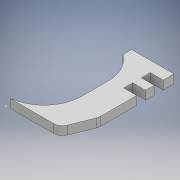
# Autodesk Inventor part: Finger
Saved by Autodesk Inventor 2017 (Build 210142000, 142)
## iProperties
Created: 2017-05-09
Part Number: Finger
Material: Generic
Document SubType Name: Modeling
Designer: s4461999
Density: 1 g/cm^3
Appearance: Default
Author: s4461999
Autodesk Inventor part; units mm, degrees
ref_plane "YZ Plane" through (0, 0, 0) normal (1, 0, 0) x (0, 1, 0)
ref_plane "XZ Plane" through (0, 0, 0) normal (0, 1, 0) x (-1, 0, 0)
ref_plane "XY Plane" through (0, 0, 0) normal (0, 0, 1) x (1, 0, 0)
sketch "Sketch1" plane through (0, 0, 0) normal (0, 0, 1) x (1, 0, 0)
  arc A0 (6.0987, 0.8622) -> (22, 22) centre (0, 22) ccw
  line L0 (22, 22) -> (22, 37)
  arc A1 (22, 37) -> (13, 54.7482) centre (0, 37) ccw
  line L1 (13, 54.7482) -> (13, 66.7482)
  line L2 (22.5, 90) -> (22.5, 66.7482)
  line L3 (22.5, 90) -> (37.5, 90)
  line L4 (13, 66.7482) -> (22.5, 66.7482)
  line L5 (2.6116, 0) -> (27.6759, 0)
  line L6 (32.3216, 3.1515) -> (37.1457, 15.2755)
  arc A2 (37.1457, 15.2755) -> (37.5, 17.1241) centre (32.5, 17.1241) ccw
  arc A3 (27.6759, 0) -> (32.3216, 3.1515) centre (27.6759, 5) ccw
  line L7 (37.5, 53.562) -> (30, 53.562)
  line L8 (30, 53.562) -> (30, 48.362)
  line L9 (30, 48.362) -> (37.5, 48.362)
  line L10 (37.5, 43.362) -> (30, 43.362)
  line L11 (30, 43.362) -> (30, 38.162)
  line L12 (30, 38.162) -> (37.5, 38.162)
  line L13 (37.5, 90) -> (37.5, 53.562)
  line L14 (37.5, 48.362) -> (37.5, 43.362)
  line L15 (37.5, 38.162) -> (37.5, 17.1241)
  line L16 (6.0987, 0.8622) -> (2.6116, 0)
  point P0 (0, 0)
  dimension "d0" = 22
  dimension "d1" = 90
  dimension "d2" = 0
  dimension "d3" = 15
  dimension "d4" = 0
  dimension "d5" = 13
  dimension "d6" = 22
  dimension "d7" = 12
  dimension "d8" = 22.5
  dimension "d10" = 90
  dimension "d11" = 37
  dimension "d12" = 5
  dimension "d13" = 12.1241
  dimension "d14" = 5.2
  dimension "d15" = 5.2
  dimension "d16" = 5
  constraints: 34 end point, 8 point on circle, 7 perpendicular, 6 tangent, 6 vertical, 4 centre point, 4 horizontal, 2 point on line, 1 equal radius, 1 parallel
  measures "d0" radius of A0
  measures "d2" horizontal distance of point (0, 0) A0.centre
  measures "d3" distance of L0.start L0.end
  measures "d4" horizontal distance of point (0, 0) A1.centre
  measures "d5" horizontal distance of A1.centre L1.start
  measures "d6" radius of A1
  measures "d7" distance of L1.start L1.end
  measures "d8" distance from line of point (0, 0) L2
  measures "d10" distance from line of point (0, 0) L3
  measures "d11" distance from line of L6 A0.centre
  measures "d12" radius of A2
  measures "d13" vertical distance of L6.start L6.end
  measures "d14" distance between parallel lines of L9 L7
  measures "d15" distance between parallel lines of L12 L10
  measures "d16" distance between parallel lines of L9 L10
sketch "Sketch2" plane through (0, 0, 0) normal (0, 0, 1) x (1, 0, 0)
  point P0 (0, 0)
extrude "Extrusion1" add sketch "Sketch1" along normal blind 5
sketch "Sketch3" plane through (0, 0, 5) normal (0, 0, 1) x (1, 0, 0)
  line L0 (22.5, 90) -> (22.5, 66.7482) projected
  line L1 (37.5, 90) -> (22.5, 90) projected
  point P0 (0, 0)
  point P1 (30, 86.5)
  point P2 (30, 68.5)
  dimension "d20" = 18
  dimension "d21" = 7.5
  dimension "d22" = 7.5
  dimension "d23" = 3.5
  measures "d20" distance of point (30, 68.5) point (30, 86.5)
  measures "d21" distance from line of point (30, 86.5) L0
  measures "d22" distance from line of L0 point (30, 68.5)
  measures "d23" distance from line of L1 point (30, 86.5)
hole "Hole1" at (30, 86.5, 5) at (30, 68.5, 5) direction (0, 0, -1) diameter 3.4 end through all
sketch "Sketch4" plane through (22.5, 66.7482, 0) normal (-1, 0, 0) x (0, 0, 1)
  line L0 (-7.9102, 0) -> (13.3435, 0)
  line L1 (13.3435, 0) -> (13.3435, 24.2425)
  line L2 (13.3435, 24.2425) -> (-7.9102, 24.2425)
  line L3 (-7.9102, 24.2425) -> (-7.9102, 0)
  line L4 (0, 0) -> (5, 0) projected
  point P0 (0, -66.7482)
  dimension "d31" = 0
  constraints: 8 end point, 2 parallel, 1 horizontal, 1 perpendicular
  measures "d31" distance between parallel lines of L4 L0
extrude "Extrusion2" cut sketch "Sketch4" against normal blind 15
sketch "Sketch5" plane through (13, 54.7482, 0) normal (-1, 0, 0) x (0, 0, 1)
  line L0 (-8.9151, 14.3214) -> (15.4889, 14.3214)
  line L1 (15.4889, 14.3214) -> (15.4889, 5)
  line L2 (15.4889, 5) -> (-8.9151, 5)
  line L3 (-8.9151, 5) -> (-8.9151, 14.3214)
  line L4 (0, 12) -> (5, 12) projected
  point P0 (0, -54.7482)
  dimension "d34" = 7
  constraints: 8 end point, 2 parallel, 1 horizontal, 1 perpendicular
  measures "d34" distance between parallel lines of L4 L2
extrude "Extrusion3" cut sketch "Sketch5" against normal blind 40
body "Solid1"
